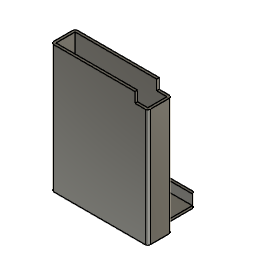
battery (Autodesk Fusion 360 design; units mm, degrees)
part number: 2025-07-05-13-13-52-023
Autodesk Fusion 360 part; units mm, degrees
sketch "Schizzo1" plane through (0, 0, 0) normal (0, 0, 1) x (1, 0, 0)
  line L0 (0, 0) -> (76, 0)
  line L1 (76, 0) -> (76, 19)
  line L2 (76, 19) -> (0, 19)
  line L3 (0, 19) -> (0, 0)
  dimension "d1" = 76
  dimension "d2" = 19
  constraint horizontal L0
  constraint vertical L1
  constraint horizontal L2
  constraint vertical L3
  constraint coincident L0.start L3.end
  measures "d1" distance of L0.start L0.end
  measures "d2" distance of L0.start L2.end
extrude "Estrusione1" add sketch "Schizzo1" along normal blind 100 makes body 1
shell "Svuotamento1" thickness 2 removed faces 1 at (25.3333, 12.6667, 100) on bodies 1
sketch "Schizzo2" plane through (76, 0, 0) normal (1, 0, 0) x (0, 1, 0)
  line L0 (0, 0) -> (19, 0)
  line L1 (19, 0) -> (19, 100)
  line L2 (19, 100) -> (0, 100)
  line L3 (0, 100) -> (0, 0)
  line L4 (0, 100) -> (19, 100)
  line L5 (19, 100) -> (19, 92)
  line L6 (19, 92) -> (0, 92)
  line L7 (0, 92) -> (0, 100)
  constraint horizontal L4
  constraint vertical L5
  constraint horizontal L6
  constraint vertical L7
  constraint coincident L1 L5.end
  constraint coincident L2.end L3.start
extrude "Estrusione2" cut sketch "Schizzo2" against normal blind 10 contours L1 L2 L3 L4 L5 L6 L7 bodies 1
sketch "Schizzo3" plane through (0, 0, 0) normal (0, 0, 1) x (1, 0, 0)
  line L0 (0, 45) -> (80, 45)
  line L1 (80, 45) -> (80, 22)
  line L2 (80, 22) -> (0, 22)
  line L3 (0, 22) -> (0, 45)
  dimension "d8" = 80
  dimension "d9" = 23
  constraint horizontal L0
  constraint vertical L1
  constraint horizontal L2
  constraint vertical L3
  measures "d8" distance of L0.start L0.end
  measures "d9" distance of L0.start L2.end
extrude "Estrusione3" add sketch "Schizzo3" along normal blind 10 separate body makes body 2
shell "Svuotamento2" thickness 2 removed faces 1 at (26.6667, 37.3333, 10) on bodies 2
sketch "Schizzo4" plane through (80, 0, 0) normal (1, 0, 0) x (0, 1, 0)
  line L0 (22, 0) -> (45, 0)
  line L1 (45, 0) -> (45, 10)
  line L2 (45, 10) -> (22, 10)
  line L3 (22, 10) -> (22, 0)
  line L4 (25, 10) -> (42.257, 10)
  line L5 (42.257, 10) -> (42.257, 2.4696)
  line L6 (42.257, 2.4696) -> (25, 2.4696)
  line L7 (25, 2.4696) -> (25, 10)
  constraint horizontal L4
  constraint vertical L5
  constraint horizontal L6
  constraint vertical L7
  constraint coincident L2 L4.start
extrude "Estrusione4" cut sketch "Schizzo4" against normal blind 20 contours L2 L4 L5 L6 L7 bodies 2
extrude "Estrusione5" cut 1 faces at (80, 23, 4.1565) along direction (-1, 0, 0) blind 12 on bodies 2 bodies 2
fillet "Raccordo1" radius 2 8 edges at (0, 19, 50) (0, 0, 50) (76, 0, 46) (76, 19, 46) (68, 22, 5) (68, 45, 5) (0, 45, 5) (0, 22, 5) on bodies 1 2
